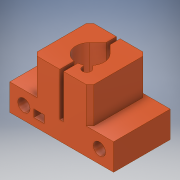
# Autodesk Inventor part: Hopper Linear Bearing Holder
Saved by Autodesk Inventor 2018 (Build 220112000, 112)
## iProperties
Created: 2013-10-19
Part Number: Hopper Linear Bearing Holder
Material: ABS Plastic
Document SubType Name: Modeling
Designer: Gabriel Smolnycki
Mass: 32.4829 g
Surface Area: 118.667 cm^2
Volume: 30.6442 cm^3
Density: 1.06 g/cm^3
Appearance: Smooth - Light Orange
Sending System: SolidWorks 2017
Last Author: Gabriel Smolnycki
Last Saved: 2017-09-14
Author: Gabriel Smolnycki
Autodesk Inventor part; units mm, degrees
ref_plane "YZ Plane" through (0, 0, 0) normal (1, 0, 0) x (0, 1, 0)
ref_plane "XY Plane" through (0, 0, 0) normal (0, 0, 1) x (1, 0, 0)
ref_plane "Work Plane1" through (0, 33, 0) normal (0, 1, 0) x (-1, 0, 0)
sketch "Sketch1" plane through (0, 33, 0) normal (0, 1, 0) x (-1, 0, 0)
  line L0 (-27.5, 15) -> (-27.5, -15)
  line L1 (-27.5, 15) -> (27.5, 15)
  line L2 (27.5, 15) -> (27.5, -15)
  line L3 (-27.5, -15) -> (27.5, -15)
  constraints: 8 end point, 2 horizontal, 2 vertical
extrude "Extrusion13" add sketch "Sketch1" against normal blind 33
sketch "Sketch2" plane through (-27.5, 33, 15) normal (0, 0, 1) x (1, 0, 0)
  line L0 (18.25, -25) -> (12.75, -25)
  line L1 (12.75, -29) -> (18.25, -29)
  line L2 (18.25, -29) -> (18.25, -25)
  line L3 (12.75, -25) -> (12.75, -29)
  constraints: 8 end point, 2 horizontal, 2 vertical
extrude "Extrusion12" cut sketch "Sketch2" against normal blind 30
sketch "Sketch3" plane through (-14.75, 4, 15) normal (0, 1, 0) x (1, 0, 0)
  arc A0 (1.5126, 6.7374) -> (3.9874, 6.7374) centre (2.75, 5.5) ccw
  line L0 (3.9874, 6.7374) -> (2.75, 7.9749)
  line L1 (2.75, 7.9749) -> (1.5126, 6.7374)
  constraints: 4 end point, 2 perpendicular, 2 point on circle, 1 centre point
extrude "Extrusion11" cut sketch "Sketch3" against normal blind 4
sketch "Sketch4" plane through (0, 0, 0) normal (0, 1, 0) x (-1, 0, 0)
  arc A0 (13.2374, -10.7374) -> (10.7626, -10.7374) centre (12, -9.5) ccw
  line L0 (13.2374, -10.7374) -> (12, -11.9749)
  line L1 (12, -11.9749) -> (10.7626, -10.7374)
  constraints: 4 end point, 2 perpendicular, 2 point on circle, 1 centre point
extrude "Extrusion10" cut sketch "Sketch4" along normal blind 4
sketch "Sketch5" plane through (-14.75, 8, 15) normal (0, -1, 0) x (1, 0, 0)
  line L0 (2.75, -7.9749) -> (3.9874, -6.7374)
  line L1 (1.5126, -6.7374) -> (2.75, -7.9749)
  arc A0 (3.9874, -6.7374) -> (1.5126, -6.7374) centre (2.75, -5.5) ccw
  constraints: 4 end point, 2 perpendicular, 2 point on circle, 1 centre point
extrude "Extrusion9" cut sketch "Sketch5" against normal blind 12
sketch "Sketch6" plane through (-14.75, 8, 15) normal (0, -1, 0) x (1, 0, 0)
  line L0 (2.75, -26.9749) -> (3.9874, -25.7374)
  line L1 (1.5126, -25.7374) -> (2.75, -26.9749)
  arc A0 (3.9874, -25.7374) -> (1.5126, -25.7374) centre (2.75, -24.5) ccw
  constraints: 4 end point, 2 perpendicular, 2 point on circle, 1 centre point
extrude "Extrusion8" cut sketch "Sketch6" against normal blind 12
sketch "Sketch7" plane through (0, 33, 0) normal (0, 1, 0) x (-1, 0, 0)
  line L0 (-4.409, 6.0942) -> (-6, 4.5032)
  arc A0 (-4.409, 6.0942) -> (-7.591, 6.0942) centre (-6, 7.6852) ccw
  line L1 (-7.591, 6.0942) -> (-6, 4.5032)
  constraints: 4 end point, 2 perpendicular, 2 point on circle, 1 centre point
extrude "Extrusion7" cut sketch "Sketch7" against normal blind 33
sketch "Sketch8" plane through (0, 33, 0) normal (0, 1, 0) x (-1, 0, 0)
  line L0 (-5.3033, -5.3033) -> (0, -10.6066)
  arc A0 (-3.7724, 7.3683) -> (-3.0726, 6.8417) centre (-3.2774, 7.2978) ccw
  arc A1 (-4.409, 6.0942) -> (-3.7724, 7.3683) centre (-6, 7.6852) ccw
  line L1 (0, -10.6066) -> (5.3033, -5.3033)
  arc A2 (5.3033, -5.3033) -> (-3.0726, 6.8417) centre (0, 0) ccw
  line L2 (-6, 4.5032) -> (-4.409, 6.0942)
  line L3 (-6.2969, 4.8001) -> (-6, 4.5032)
  arc A3 (-6.2348, 4.1686) -> (-6.2969, 4.8001) centre (-6.6504, 4.4466) ccw
  arc A4 (-6.2348, 4.1686) -> (-5.3033, -5.3033) centre (0, 0) ccw
  constraints: 10 point on circle, 8 end point, 5 centre point, 3 perpendicular, 1 parallel
extrude "Extrusion6" cut sketch "Sketch8" against normal blind 24 draft 0
sketch "Sketch9" plane through (0, 33, 0) normal (0, 1, 0) x (-1, 0, 0)
  line L0 (0, -10.6066) -> (-1, -9.6066)
  line L1 (1, -9.6066) -> (0, -10.6066)
  line L2 (-1, -9.6066) -> (-1, -15)
  line L3 (-1, -15) -> (1, -15)
  line L4 (1, -9.6066) -> (1, -15)
  constraints: 10 end point, 2 equal length, 2 vertical, 1 horizontal, 1 perpendicular
extrude "Extrusion5" cut sketch "Sketch9" against normal blind 23 draft 0
sketch "Sketch10" plane through (0, 33, 0) normal (0, 1, 0) x (-1, 0, 0)
  line L0 (-1, 15) -> (1, 15)
  arc A0 (1, 7.433) -> (-1, 7.433) centre (0, 0) ccw
  line L1 (-1, 15) -> (-1, 7.433)
  line L2 (1, 15) -> (1, 7.433)
  constraints: 6 end point, 2 point on circle, 2 vertical, 1 centre point, 1 horizontal, 1 parallel
extrude "Extrusion4" cut sketch "Sketch10" against normal blind 23 draft 0
sketch "Sketch11" plane through (0, 33, 0) normal (0, 1, 0) x (-1, 0, 0)
  line L0 (15, -13) -> (13, -15)
  line L1 (13, 15) -> (27.5, 15)
  line L2 (15, 13) -> (15, -13)
  line L3 (27.5, 15) -> (27.5, -15)
  line L4 (13, 15) -> (15, 13)
  line L5 (13, -15) -> (27.5, -15)
  constraints: 12 end point, 2 equal length, 2 horizontal, 2 vertical, 1 perpendicular
extrude "Extrusion3" cut sketch "Sketch11" against normal blind 19 draft 0
sketch "Sketch12" plane through (0, 33, 0) normal (0, 1, 0) x (-1, 0, 0)
  line L0 (-27.5, 15) -> (-13, 15)
  line L1 (-13, -15) -> (-15, -13)
  line L2 (-15, 13) -> (-13, 15)
  line L3 (-27.5, -15) -> (-13, -15)
  line L4 (-27.5, 15) -> (-27.5, -15)
  line L5 (-15, 13) -> (-15, -13)
  constraints: 12 end point, 2 equal length, 2 horizontal, 2 vertical, 1 perpendicular
extrude "Extrusion2" cut sketch "Sketch12" against normal blind 19 draft 0
sketch "Sketch13" plane through (0, 9, 0) normal (0, 1, 0) x (1, 0, 0)
  line L0 (0, 7.0711) -> (3.5355, 3.5355)
  arc A0 (-3.5355, 3.5355) -> (3.5355, 3.5355) centre (0, 0) ccw
  line L1 (-3.5355, 3.5355) -> (0, 7.0711)
  constraints: 4 end point, 2 perpendicular, 2 point on circle, 1 centre point
extrude "Extrusion1" cut sketch "Sketch13" against normal blind 9
hole "Hole2" at (20, 7, 15) direction (0, 0, -1) diameter 6.5 depth 30 tip angle 118
sketch "Sketch14" plane through (-27.5, 0, 15) normal (0, 0, 1) x (1, 0, 0)
  point P0 (47.5, 7)
hole "Hole1" at (-20, 7, 15) direction (0, 0, -1) diameter 6.5 depth 30 tip angle 118
sketch "Sketch15" plane through (-27.5, 0, 15) normal (0, 0, 1) x (1, 0, 0)
  point P0 (7.5, 7)
body "Solid3"
